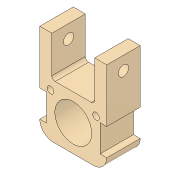
# Autodesk Inventor part: Smaller Needle Bearing Mount
Saved by Autodesk Inventor 2018.3 (Build 223284000, 284)
## iProperties
Created: 2019-03-20
Part Number: Smaller Needle Bearing Mount
Material: Polyethylene, High Density
Document SubType Name: Modeling
Designer: aye06091
Mass: 9.92488 g
Surface Area: 57.4995 cm^2
Volume: 10.4253 cm^3
Density: 0.952 g/cm^3
Appearance: Smooth - Off-White
Author: aye06091
Autodesk Inventor part; units mm, degrees
ref_plane "YZ Plane" through (0, 0, 0) normal (1, 0, 0) x (0, 1, 0)
ref_plane "XZ Plane" through (0, 0, 0) normal (0, 1, 0) x (-1, 0, 0)
ref_plane "XY Plane" through (0, 0, 0) normal (0, 0, 1) x (1, 0, 0)
sketch "Sketch1" plane through (0, 0, 0) normal (0, 0, 1) x (1, 0, 0)
  line L0 (0, -3.175) -> (31.75, -3.175)
  line L1 (31.75, -3.175) -> (31.75, -28.575)
  line L2 (31.75, -28.575) -> (0, -28.575)
  line L3 (0, -28.575) -> (0, -3.175)
  line L4 (0, -3.175) -> (5.715, -3.175)
  line L5 (5.715, -3.175) -> (5.715, 15.875)
  line L6 (5.715, 15.875) -> (0, 15.875)
  line L7 (0, 15.875) -> (0, -3.175)
  line L8 (26.035, -3.175) -> (31.75, -3.175)
  line L9 (31.75, -3.175) -> (31.75, 15.875)
  line L10 (31.75, 15.875) -> (26.035, 15.875)
  line L11 (26.035, 15.875) -> (26.035, -3.175)
  point P0 (0, 0)
  dimension "d0" = 25.4
  dimension "d1" = 5.715
  dimension "d2" = 5.715
  dimension "d3" = 19.05
  dimension "d4" = 31.75
  dimension "d24" = 20.32
  constraints: 24 end point, 6 parallel, 5 point on line, 3 horizontal, 3 perpendicular
  measures "d0" distance of L2.end L0.start
  measures "d1" distance between parallel lines of L9 L11
  measures "d2" distance of L5.end L6.end
  measures "d3" distance of L6.end L4.start
  measures "d4" distance between parallel lines of L1 L3
  measures "d24" distance between parallel lines of L11 L5
extrude "Extrusion1" add sketch "Sketch1" against normal blind 15.875
sketch "Sketch2" plane through (0, 0, 0) normal (0, 0, 1) x (1, 0, 0)
  line L0 (31.75, -28.575) -> (0, -28.575) projected
  circle A0 centre (15.875, -15.875) radius 8.7439
  dimension "d10" = 17.4879
  dimension "d13" = 12.7
  constraints: 1 centre point
  measures "d10" diameter of A0
  measures "d13" distance from line of L0 A0.centre
extrude "Extrusion2" cut sketch "Sketch2" against normal blind 15.875
sketch "Sketch3" plane through (31.75, -3.175, 0) normal (1, 0, 0) x (0, 0, -1)
  line L0 (0, 19.05) -> (15.875, 19.05) projected
  line L1 (-0.1272, 19.05) -> (15.7478, 19.05)
  circle A0 centre (7.9375, 12.7) radius 2.4447
  dimension "d16" = 4.8895
  dimension "d17" = 6.35
  dimension "d18" = 0
  constraints: 2 end point, 1 centre point
  measures "d16" diameter of A0
  measures "d17" distance from line of L1 A0.centre
  measures "d18" distance between parallel lines of L1 L0
extrude "Extrusion3" cut sketch "Sketch3" against normal through all
fillet "Fillet1" radius 1.5875 2 edges at (5.715, -3.175, -7.9375) (26.035, -3.175, -7.9375)
fillet "Fillet3" radius 6.35 2 edges at (0, -28.575, -7.9375) (31.75, -28.575, -7.9375)
sketch "Sketch4" plane through (0, 0, 0) normal (0, 0, 1) x (1, 0, 0)
  line L0 (31.75, 15.875) -> (31.75, -22.225) projected
  line L1 (0, -22.225) -> (0, 15.875) projected
  circle A0 centre (15.875, -15.875) radius 8.7439 projected
  circle A1 centre (5.08, -7.7365) radius 1.6002
  circle A2 centre (26.67, -7.7365) radius 1.6002
  point P0 (0, 0)
  dimension "d25" = 3.2004
  dimension "d26" = 3.175
  dimension "d27" = 5.08
  dimension "d28" = 3.175
  dimension "d29" = 5.08
  dimension "d32" = 3.2004
  constraints: 2 centre point
  measures "d25" diameter of A1
  measures "d27" distance from line of L1 A1.centre
  measures "d29" distance from line of L0 A2.centre
  measures "d32" diameter of A2
extrude "Extrusion4" cut sketch "Sketch4" against normal blind 25.4 contours A1 | A2
sketch "Sketch5" plane through (0, 0, 0) normal (0, 0, 1) x (1, 0, 0)
  line L0 (31.75, 15.875) -> (31.75, -22.225) projected
  line L1 (0, -22.225) -> (0, 15.875) projected
  line L2 (0, -22.2885) -> (3.175, -22.2885)
  line L3 (3.175, -22.2885) -> (3.175, -9.4615)
  line L4 (3.175, -9.4615) -> (0, -9.4615)
  line L5 (0, -9.4615) -> (0, -22.2885)
  line L6 (31.75, -9.4615) -> (28.575, -9.4615)
  line L7 (28.575, -9.4615) -> (28.575, -22.2885)
  line L8 (28.575, -22.2885) -> (31.75, -22.2885)
  line L9 (31.75, -22.2885) -> (31.75, -9.4615)
  circle A0 centre (15.875, -15.875) radius 8.7439 projected
  point P0 (0, 0)
  point P1 (3.175, -15.875)
  dimension "d33" = 12.827
  dimension "d34" = 3.175
  dimension "d35" = 3.175
  dimension "d41" = 0
  constraints: 16 end point, 4 parallel, 4 point on line, 2 horizontal, 2 perpendicular, 1 midpoint
  measures "d33" distance of L2.end L3.end
  measures "d34" distance of L2.start L2.end
  measures "d35" distance of L7.end L8.end
  measures "d41" vertical distance of A0.centre point (3.175, -15.875)
extrude "Extrusion5" cut sketch "Sketch5" against normal blind 25.4 contours L0 L9 L8 L7 L6 | L1 L4 L3 L2 L5
body "Solid1"
